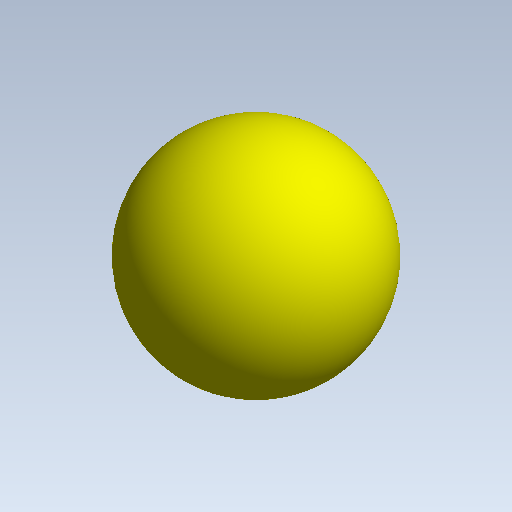
# Autodesk Inventor part: W 627/4-2ZS_PART3
Saved by Autodesk Inventor 2021 (Build 250183000, 183)
## iProperties
Part Number: W 627/4-2ZS_PART3
Material: Allgemein
Catalog Web Link: www.cadenas.de
Description: -Deep groove ball bearings
Vendor: SKF
Document SubType Name: Modeling
Designer: partserver
Manufacturer: SKF
Mass: 0.000268083 g
Surface Area: 0.0201062 cm^2
Volume: 0.000268083 cm^3
Density: 1 g/cm^3
Appearance: PSOLRGB-192-192-192
Category: PARTsolutions
Company: SKF
PSOL_IDENT_0: {$CADENAS_DATA\23d-libs\skf\bearings_units_and_housings\ball_bearings\deep_groove_ball_bearings\bb1_
PSOL_IDENT_1: 001_101.prj},201 {VTYP=3D},{NB=W 627/4-2ZS_PART3},{LINA=W 627/4-2ZS_PART3},{NN=BB1_001_101_PART3},{N
PSOL_IDENT_2: OPRJ=TRUE},{DATE=19.12.2019 14:34:47},{GEOMDATE=18.12.2019 13:53:11},{VERSION=},{LINEID=18320},{WBVA
PSOL_IDENT_3: R=},{WBNUMERIC=}  {NB=W 627/4-2ZS_PART3},{LINA=W 627/4-2ZS_PART3},{KT=DUMMY},{PRODUCTID=},{DESIGNATI
PSOL_IDENT_4: ON=W 627/4-2ZS},{DD=4.000},{D=7.000},{B=2.500},{C=0.000},{DD1=4.80},{DD2=0.00},{D1=0.00},{D2=6.30},{
PSOL_IDENT_5: D3=0.000},{D4=0.000},{HH=MIN},{BB=0.000},{FF=0.00},{R0MAX=MIN},{R0=MIN},{R12=0.10},{PITCH=5.40},{DW=
PSOL_IDENT_6: 0.800},{DDAMIN=4.600},{DDAMAX=4.700},{DDBMIN=MIN},{DDBMAX=MIN},{DBMIN=MIN},{DAMAX=6.400},{BBAMIN=MIN
PSOL_IDENT_7: },{CAMAX=MIN},{RAMAX=0.100},{LOAD1=0.143},{LOAD2=0.053},{LOAD3=0.002},{SPEED1=150000},{SPEED2=75000}
PSOL_IDENT_8: ,{KR=0.015},{F0=7.600},{Z=11},{II=1},{MASS=0.000},{BEARING=W 627/4-2ZS},{RING=},{HELP=0.532},{HELP2=
PSOL_IDENT_9: 0.350},{DD1ALG=2.400},{YALG=2.400},{PITCH1=5.400},{DW1=0.800},{YALG1=2.968},{HALG1=0.532},{SH=2.400}
PSOL_IDENT_10: ,{CU=0.340},{DESIGN=dgbbw2z},{HALG=0.4},{B1=0},{SHIELDHELP=2}
NB: W 627/4-2ZS_PART3
NT: Deep groove ball bearings
NBSYN: $DESIGNATION._PART3
LINA: W 627/4-2ZS_PART3
CATALOG: SKF
SUPPLIER: SKF
ARTICLENO: W 627/4-2ZS_PART3
BOMINFO: W 627/4-2ZS_PART3
CREATOR: CADENAS GmbH
Title: W 627/4-2ZS_PART3
Author: Cadenas PARTsolutions
Comments: Deep groove ball bearings
Autodesk Inventor part; units mm, degrees
ref_plane "YZ Plane" through (0, 0, 0) normal (1, 0, 0) x (0, 1, 0)
ref_plane "XZ Plane" through (0, 0, 0) normal (0, 1, 0) x (-1, 0, 0)
ref_plane "XY Plane" through (0, 0, 0) normal (0, 0, 1) x (1, 0, 0)
sketch "Sketch_6" plane through (0, 0, 0) normal (0, 0, 1) x (1, 0, 0)
  line L0 (1.65, 2.7) -> (0.85, 2.7)
  arc A0 (1.65, 2.7) -> (0.85, 2.7) centre (1.25, 2.7) ccw
  line L1 (1.65, 2.7) -> (0.85, 2.7)
  dimension "d0" = 360
  constraints: 4 end point, 2 point on circle, 1 centre point
revolve "Revolution1" add sketch "Sketch_6" angle 360 about axis through (1.65, 2.7, 0) along (1, 0, 0)
body "Solid1"
